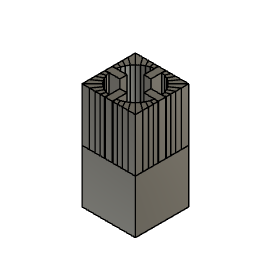
slotted_circle_hole_V2 v2 (Autodesk Fusion 360 design; units mm, degrees)
Autodesk Fusion 360 part; units mm, degrees
note: some values were not read from the file. Chosen so that the rebuilt part matches the saved one: which bodies a step acts on; which face or edge a step refers to. Set by a fixed rule: which sketch regions a step uses.
sketch "Sketch1" plane through (0, 0, 0) normal (0, 0, 1) x (1, 0, 0)
  line L0 (15, 15) -> (-15, 15)
  line L1 (-15, 15) -> (-15, -15)
  line L2 (-15, -15) -> (15, -15)
  line L3 (15, -15) -> (15, 15)
  line L4 (15, 15) -> (-15, -15) construction
  line L5 (-15, 15) -> (15, -15) construction
  circle A0 centre (0, 0) radius 13
  circle A1 centre (0, 0) radius 12.5
  line L6 (0, 0) -> (0, 12.5)
  line L7 (2, 6.75) -> (-2, 6.75)
  line L8 (-2, 6.75) -> (-2, 18.25)
  line L9 (-2, 18.25) -> (2, 18.25)
  line L10 (2, 18.25) -> (2, 6.75)
  line L11 (2, 6.75) -> (-2, 18.25) construction
  line L12 (-2, 6.75) -> (2, 18.25) construction
  line L13 (-6.75, 2) -> (-6.75, -2)
  line L14 (-6.75, -2) -> (-18.25, -2)
  line L15 (-18.25, 2) -> (-6.75, 2)
  line L16 (-15, 15) -> (-15, -15)
  line L17 (-2, -6.75) -> (2, -6.75)
  line L18 (2, -6.75) -> (2, -18.25)
  line L19 (-2, -18.25) -> (-2, -6.75)
  line L20 (-15, -15) -> (15, -15)
  line L21 (6.75, -2) -> (6.75, 2)
  line L22 (6.75, 2) -> (18.25, 2)
  line L23 (18.25, -2) -> (6.75, -2)
  line L24 (15, -15) -> (15, 15)
  point P0 (0, 12.5)
  dimension "d1" = 30
  dimension "d2" = 30
  dimension "d3" = 26
  dimension "d4" = 25
  dimension "d5" = 4
  dimension "d6" = 5.75
  dimension "d8" = 360
  constraint horizontal L0
  constraint perpendicular L0 L1
  constraint parallel L0 L2
  constraint parallel L1 L3
  constraint coincident L4 A0.centre
  constraint coincident L5 A0.centre
  constraint coincident A0.centre A1.centre
  constraint concentric A0 A1
  constraint coincident A1 P0
  constraint vertical L6
  constraint horizontal L7
  constraint perpendicular L7 L8
  constraint parallel L7 L9
  constraint parallel L8 L10
  constraint coincident L11 P0
  constraint coincident L12 P0
  constraint coincident P0 L6.end
  measures "d1" distance of L0.end L1.end L17
  measures "d2" distance of L1.end L2.end
  measures "d3" diameter of A0
  measures "d4" diameter of A1
  measures "d5" distance of L8.end L9.end
  measures "d6" distance of L7 P0
extrude "Extrude1" add sketch "Sketch1" against normal blind 30 contours L0 L3 A0 L10 L22 L24 | L0 A0 L8 L10 | L3 A0 L22 L23 L24 | L0 L1 A0 L8 L15 L16 | A0 A1 L8 L10 | L2 L3 A0 L18 L20 L23 L24 | A0 A1 L22 L23 | A1 L6 L7 L10 | A1 L21 L22 L23 | L1 A0 L14 L15 L16 | A0 A1 L14 L15 | A1 L6 L7 L8 | L2 A0 L18 L19 L20 | A0 A1 L18 L19 | L1 L2 A0 L14 L16 L19 L20 | A1 L13 L14 L15 | A1 L17 L18 L19 makes body 1
sketch "Sketch2" plane through (0, 0, -30) normal (0, 0, -1) x (1, 0, 0)
  arc A0 (12.8452, 2) -> (2, 12.8452) centre (0, 0) ccw
  line L0 (12.8452, 2) -> (6.75, 2)
  line L1 (6.75, 2) -> (6.75, -2)
  line L2 (6.75, -2) -> (12.8452, -2)
  arc A1 (2, -12.8452) -> (12.8452, -2) centre (0, 0) ccw
  line L3 (2, -12.8452) -> (2, -6.75)
  line L4 (2, -6.75) -> (-2, -6.75)
  line L5 (-2, -6.75) -> (-2, -12.8452)
  arc A2 (-12.8452, -2) -> (-2, -12.8452) centre (0, 0) ccw
  line L6 (-12.8452, -2) -> (-6.75, -2)
  line L7 (-6.75, -2) -> (-6.75, 2)
  line L8 (-6.75, 2) -> (-12.8452, 2)
  arc A3 (-2, 12.8452) -> (-12.8452, 2) centre (0, 0) ccw
  line L9 (-2, 12.8452) -> (-2, 6.75)
  line L10 (-2, 6.75) -> (2, 6.75)
  line L11 (2, 6.75) -> (2, 12.8452)
  line L12 (-15, -15) -> (15, -15)
  line L13 (15, -15) -> (15, 15)
  line L14 (15, 15) -> (-15, 15)
  line L15 (-15, 15) -> (-15, -15)
extrude "Extrude2" add sketch "Sketch2" along normal blind 30 contours A0 L0 L1 L2 A1 L3 L4 L5 A2 L6 L7 L8 A3 L9 L10 L11 | L12 L13 L14 L15 bodies 1
move_body "Move1" bodies 1 to x (1, 0, 0) y (0, 1, 0) z (0, 0, 1) at (0, 0, 30)
split "Split1" by plane through (0, 0, 0) normal (0, 0, 1) bodies 1 makes body 2 at (15, -5, 20)
split "Split2" by plane through (-12.339, -2, 30) normal (0, -1, 0) and through (-12.339, 2, 30) normal (0, 1, 0) bodies 2 makes body 3 at (-5, -15, 10) makes body 4 at (-10.8135, -2, 10) makes body 5 at (5, 15, 10)
split "Split3" by plane through (2, 12.339, 30) normal (1, 0, 0) and through (-2, 12.339, 30) normal (-1, 0, 0) bodies 5 makes body 6 at (12.7378, 2.5979, 20) makes body 7 at (-10.5666, 7.5727, 10)
split "Split4" by plane through (-2, -12.339, 30) normal (-1, 0, 0) and through (2, -12.339, 30) normal (1, 0, 0) bodies 3 makes body 8 at (-3.1902, -12.6025, 10) makes body 9 at (12.7378, -2.5979, 10)
sketch "Sketch3" plane through (0, 0, 30) normal (0, 0, 1) x (-1, 0, 0)
  line L0 (2, -12.8452) -> (2, -15)
  line L1 (2, -15) -> (15, -15)
  line L2 (15, -15) -> (15, -2)
  line L3 (15, -2) -> (12.8452, -2)
  arc A0 (2, -12.8452) -> (12.8452, -2) centre (0, 0) ccw
  line L4 (0, 0) -> (15, -15)
  line L5 (0, 0) -> (17.1618, -12.4688)
  line L6 (0, 0) -> (18.9011, -9.6306)
  line L7 (0, 0) -> (20.175, -6.5552)
  line L8 (0, 0) -> (20.952, -3.3185)
  line L9 (0, 0) -> (21.2132, 0)
  line L10 (0, 0) -> (20.952, 3.3185)
  line L11 (0, 0) -> (20.175, 6.5552)
  line L12 (0, 0) -> (18.9011, 9.6306)
  line L13 (0, 0) -> (17.1618, 12.4688)
  line L14 (0, 0) -> (15, 15)
  line L15 (0, 0) -> (12.4688, 17.1618)
  line L16 (0, 0) -> (9.6306, 18.9011)
  line L17 (0, 0) -> (6.5552, 20.175)
  line L18 (0, 0) -> (3.3185, 20.952)
  line L19 (0, 0) -> (0, 21.2132)
  line L20 (0, 0) -> (-3.3185, 20.952)
  line L21 (0, 0) -> (-6.5552, 20.175)
  line L22 (0, 0) -> (-9.6306, 18.9011)
  line L23 (0, 0) -> (-12.4688, 17.1618)
  line L24 (0, 0) -> (-15, 15)
  line L25 (0, 0) -> (-17.1618, 12.4688)
  line L26 (0, 0) -> (-18.9011, 9.6306)
  line L27 (0, 0) -> (-20.175, 6.5552)
  line L28 (0, 0) -> (-20.952, 3.3185)
  line L29 (0, 0) -> (-21.2132, 0)
  line L30 (0, 0) -> (-20.952, -3.3185)
  line L31 (0, 0) -> (-20.175, -6.5552)
  line L32 (0, 0) -> (-18.9011, -9.6306)
  line L33 (0, 0) -> (-17.1618, -12.4688)
  line L34 (0, 0) -> (-15, -15)
  line L35 (0, 0) -> (-12.4688, -17.1618)
  line L36 (0, 0) -> (-9.6306, -18.9011)
  line L37 (0, 0) -> (-6.5552, -20.175)
  line L38 (0, 0) -> (-3.3185, -20.952)
  line L39 (0, 0) -> (0, -21.2132)
  line L40 (0, 0) -> (3.3185, -20.952)
  line L41 (0, 0) -> (6.5552, -20.175)
  line L42 (0, 0) -> (9.6306, -18.9011)
  line L43 (0, 0) -> (12.4688, -17.1618)
  dimension "d15" = 360
  constraint coincident A0.centre L4.start
  constraint coincident L1.end L2.start
ref_plane "WorkPlane2" through (0, -10.6066, 30) normal (-1, 0, 0) x (0, -1, 0)
ref_plane "WorkPlane3" through (-1.6592, -10.476, 30) normal (-0.987688, 0.156434, 0) x (-0.156434, -0.987688, 0)
ref_plane "WorkPlane4" through (-3.2776, -10.0875, 30) normal (-0.951057, 0.309017, 0) x (-0.309017, -0.951057, 0)
ref_plane "WorkPlane5" through (-4.8153, -9.4506, 30) normal (-0.891007, 0.45399, 0) x (-0.45399, -0.891007, 0)
ref_plane "WorkPlane6" through (-6.2344, -8.5809, 30) normal (-0.809017, 0.587785, 0) x (-0.587785, -0.809017, 0)
ref_plane "WorkPlane7" through (-7.5, -7.5, 30) normal (-0.707107, 0.707107, 0) x (-0.707107, -0.707107, 0)
ref_plane "WorkPlane8" through (-8.5809, -6.2344, 30) normal (-0.587785, 0.809017, 0) x (-0.809017, -0.587785, 0)
ref_plane "WorkPlane9" through (-9.4506, -4.8153, 30) normal (-0.45399, 0.891007, 0) x (-0.891007, -0.45399, 0)
ref_plane "WorkPlane10" through (-10.0875, -3.2776, 30) normal (-0.309017, 0.951057, 0) x (-0.951057, -0.309017, 0)
ref_plane "WorkPlane11" through (-10.476, -1.6592, 30) normal (-0.156434, 0.987688, 0) x (-0.987688, -0.156434, 0)
ref_plane "WorkPlane12" through (-10.6066, 0, 30) normal (0, 1, 0) x (-1, 0, 0)
ref_plane "WorkPlane13" through (-10.476, 1.6592, 30) normal (0.156434, 0.987688, 0) x (-0.987688, 0.156434, 0)
ref_plane "WorkPlane14" through (-10.0875, 3.2776, 30) normal (0.309017, 0.951057, 0) x (-0.951057, 0.309017, 0)
ref_plane "WorkPlane15" through (-9.4506, 4.8153, 30) normal (0.45399, 0.891007, 0) x (-0.891007, 0.45399, 0)
ref_plane "WorkPlane16" through (-8.5809, 6.2344, 30) normal (0.587785, 0.809017, 0) x (-0.809017, 0.587785, 0)
ref_plane "WorkPlane17" through (-7.5, 7.5, 30) normal (0.707107, 0.707107, 0) x (-0.707107, 0.707107, 0)
ref_plane "WorkPlane18" through (-6.2344, 8.5809, 30) normal (0.809017, 0.587785, 0) x (-0.587785, 0.809017, 0)
ref_plane "WorkPlane19" through (-4.8153, 9.4506, 30) normal (0.891007, 0.45399, 0) x (-0.45399, 0.891007, 0)
ref_plane "WorkPlane20" through (-3.2776, 10.0875, 30) normal (0.951057, 0.309017, 0) x (-0.309017, 0.951057, 0)
ref_plane "WorkPlane21" through (-1.6592, 10.476, 30) normal (0.987688, 0.156434, 0) x (-0.156434, 0.987688, 0)
ref_plane "WorkPlane22" through (0, 10.6066, 30) normal (1, 0, 0) x (0, 1, 0)
split "Split5" by curves path "Sketch3" along L18 bodies 8 makes body 10 at (-2.6301, -12.7312, 10)
split "Split6" by plane through (-3.2776, -10.0875, 30) normal (-0.951057, 0.309017, 0) bodies 10 makes body 11 at (-9.0814, -9.302, 10)
split "Split7" by plane through (-4.8153, -9.4506, 30) normal (-0.891007, 0.45399, 0) bodies 11 makes body 12 at (-15, -10.6667, 10)
split "Split8" by plane through (-6.2344, -8.5809, 30) normal (-0.809017, 0.587785, 0) bodies 12 makes body 13 at (-15, -10.6667, 10)
split "Split9" by plane through (-7.5, -7.5, 30) normal (-0.707107, 0.707107, 0) bodies 13 makes body 14 at (-15, -10.6667, 10)
split "Split10" by plane through (-8.5809, -6.2344, 30) normal (-0.587785, 0.809017, 0) bodies 14 makes body 15 at (-15, -7.9321, 20)
split "Split11" by plane through (-9.4506, -4.8153, 30) normal (-0.45399, 0.891007, 0) bodies 15 makes body 16 at (-15, -5.7619, 20)
split "Split12" by plane through (-10.0875, -3.2776, 30) normal (-0.309017, 0.951057, 0) bodies 16 makes body 17 at (-15, -2.9579, 20)
split "Split13" by plane through (-10.476, -1.6592, 30) normal (-0.156434, 0.987688, 0) bodies 17 makes body 18 at (-13.5635, -2, 10)
split "Split14" by plane through (-10.476, 1.6592, 30) normal (0.156434, 0.987688, 0) bodies 7 makes body 19 at (-4.9142, 12.0354, 10)
split "Split15" by plane through (-10.0875, 3.2776, 30) normal (0.309017, 0.951057, 0) bodies 19 makes body 20 at (-6.4803, 11.2697, 10)
split "Split16" by plane through (-9.4506, 4.8153, 30) normal (0.45399, 0.891007, 0) bodies 20 makes body 21 at (-6.3333, 15, 10)
split "Split17" by plane through (-8.5809, 6.2344, 30) normal (0.587785, 0.809017, 0) bodies 21 makes body 22 at (-6.3333, 15, 10)
split "Split18" by plane through (-7.5, 7.5, 30) normal (0.707107, 0.707107, 0) bodies 22 makes body 23 at (-6.3333, 15, 10)
split "Split19" by plane through (-6.2344, 8.5809, 30) normal (0.809017, 0.587785, 0) bodies 23 makes body 24 at (-4.966, 15, 20)
split "Split20" by plane through (-4.8153, 9.4506, 30) normal (0.891007, 0.45399, 0) bodies 24 makes body 25 at (-3.881, 15, 20)
split "Split21" by plane through (-3.2776, 10.0875, 30) normal (0.951057, 0.309017, 0) bodies 25 makes body 26 at (-2.9579, 15, 20)
split "Split22" by plane through (-1.6592, 10.476, 30) normal (0.987688, 0.156434, 0) bodies 26 makes body 27 at (-2, 13.5635, 10)
split "Split23" by plane through (-1.6592, -10.476, 30) normal (-0.987688, 0.156434, 0) bodies 6 makes body 28 at (2, 13.5635, 10)
split "Split24" by plane through (-3.2776, -10.0875, 30) normal (-0.951057, 0.309017, 0) bodies 6 makes body 29 at (3.2084, 15, 10)
split "Split25" by plane through (-4.8153, -9.4506, 30) normal (-0.891007, 0.45399, 0) bodies 6 makes body 30 at (4.5883, 14.1212, 20)
split "Split26" by plane through (-6.2344, -8.5809, 30) normal (-0.809017, 0.587785, 0) bodies 6 makes body 31 at (7.0625, 13.861, 20)
split "Split27" by plane through (-7.5, -7.5, 30) normal (-0.707107, 0.707107, 0) bodies 6 makes body 32 at (9.8125, 13.5057, 10)
split "Split28" by plane through (-8.5809, -6.2344, 30) normal (-0.587785, 0.809017, 0) bodies 6 makes body 33 at (11.1283, 11.1283, 20)
split "Split29" by plane through (-9.4506, -4.8153, 30) normal (-0.45399, 0.891007, 0) bodies 6 makes body 34 at (13.5057, 9.8125, 10)
split "Split30" by plane through (-10.0875, -3.2776, 30) normal (-0.309017, 0.951057, 0) bodies 6 makes body 35 at (12.7221, 6.4822, 10)
split "Split31" by plane through (-10.476, -1.6592, 30) normal (-0.156434, 0.987688, 0) bodies 6 makes body 36 at (13.2425, 4.3027, 10)
split "Split32" by plane through (-10.476, 1.6592, 30) normal (0.156434, 0.987688, 0) bodies 9 makes body 37 at (13.5635, -2, 20)
split "Split33" by plane through (-10.0875, 3.2776, 30) normal (0.309017, 0.951057, 0) bodies 9 makes body 38 at (15, -3.2084, 10)
split "Split34" by plane through (-9.4506, 4.8153, 30) normal (0.45399, 0.891007, 0) bodies 9 makes body 39 at (14.1212, -4.5883, 20)
split "Split35" by plane through (-8.5809, 6.2344, 30) normal (0.587785, 0.809017, 0) bodies 9 makes body 40 at (13.861, -7.0625, 20)
split "Split36" by plane through (-7.5, 7.5, 30) normal (0.707107, 0.707107, 0) bodies 9 makes body 41 at (13.5057, -9.8125, 20)
split "Split37" by plane through (-6.2344, 8.5809, 30) normal (0.809017, 0.587785, 0) bodies 9 makes body 42 at (13.0641, -13.0641, 10)
split "Split38" by plane through (-4.8153, 9.4506, 30) normal (0.891007, 0.45399, 0) bodies 9 makes body 43 at (9.8125, -13.5057, 20)
split "Split39" by plane through (-3.2776, 10.0875, 30) normal (0.951057, 0.309017, 0) bodies 9 makes body 44 at (7.0625, -13.861, 10)
split "Split40" by plane through (-1.6592, 10.476, 30) normal (0.987688, 0.156434, 0) bodies 9 makes body 45 at (4.5883, -14.1212, 20)
